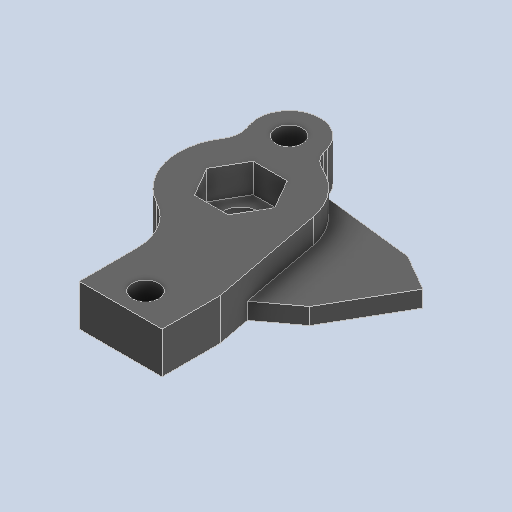
# Autodesk Inventor part: screw_lift_under
Saved by Autodesk Inventor 2024.1 (Build 281209000, 209)
## iProperties
Created: 2025-01-18
Part Number: screw_lift_under
Material: 一般
Document SubType Name: Modeling
Designer: hibik
Density: 1 g/cm^3
Appearance: 既定
Author: hibik
Autodesk Inventor part; units mm, degrees
ref_plane "YZ Plane" through (0, 0, 0) normal (1, 0, 0) x (0, 1, 0)
ref_plane "XZ Plane" through (0, 0, 0) normal (0, 1, 0) x (-1, 0, 0)
ref_plane "XY Plane" through (0, 0, 0) normal (0, 0, 1) x (1, 0, 0)
sketch "スケッチ1" plane through (0, 0, 0) normal (0, 1, 0) x (-1, 0, 0)
  line L0 (0, 0) -> (-19.1969, -33.25)
  line L1 (-19.1969, -33.25) -> (-10.9697, -38)
  line L2 (-10.9697, -38) -> (10.656, -38)
  line L3 (23.0438, 0) -> (-50.7627, 0) projected
  circle A0 centre (0, -50.5) radius 12.5
  line L4 (-19.1969, -33.25) -> (-30, -51.9615)
  line L5 (-30, -51.9615) -> (-40.219, -46.0616) construction
  line L6 (-30, -51.9615) -> (-24.5152, -61.4615)
  line L7 (-10.9697, -38) -> (-24.5152, -61.4615)
  line L8 (-24.5152, -61.4615) -> (-14.7652, -44.574)
  line L9 (-14.7652, -44.574) -> (-9.2226, -47.774)
  line L10 (-9.2226, -47.774) -> (-18.9726, -64.6615)
  line L11 (-18.9726, -64.6615) -> (-24.5152, -61.4615)
  line L12 (-10, -38) -> (-10, -31)
  line L13 (-10, -31) -> (0, -31)
  line L14 (0, -31) -> (0, -38)
  line L15 (2.0496, -46.95) -> (4.0992, -50.5)
  line L16 (4.0992, -50.5) -> (2.0496, -54.05)
  line L17 (2.0496, -54.05) -> (-2.0496, -54.05)
  line L18 (-2.0496, -54.05) -> (-4.0992, -50.5)
  line L19 (-4.0992, -50.5) -> (-2.0496, -46.95)
  line L20 (-2.0496, -46.95) -> (2.0496, -46.95)
  circle A1 centre (0, -50.5) radius 7.5
  arc A2 (0, -38) -> (3.5294, -43.8824) centre (6.6667, -38) ccw
  line L21 (-10, -38) -> (-7.3691, -51.8953)
  line L22 (-14.2226, -56.4343) -> (-18.5527, -53.9343)
  line L23 (-18.5527, -53.9343) -> (-13.5527, -45.274)
  line L24 (-13.5527, -45.274) -> (-9.2226, -47.774)
  line L25 (-9.2226, -47.774) -> (-14.2226, -56.4343)
  line L26 (-13.5527, -45.274) -> (-9.2294, -42.0698)
  line L27 (-14.2226, -56.4343) -> (-0.8456, -57.9522)
  dimension "d0" = 38
  dimension "d1" = 60
  dimension "d2" = 9.5
  dimension "d3" = 25
  dimension "d4" = 60
  dimension "d5" = 60
  dimension "d6" = 19.5
  dimension "d7" = 6.4
  dimension "d8" = 10
  dimension "d9" = 7
  dimension "d10" = 7.1
  dimension "d11" = 15
  dimension "d12" = 5
  dimension "d13" = 10
  constraints: 54 end point, 7 point on circle, 5 parallel, 5 perpendicular, 5 point on line, 5 tangent, 3 centre point, 3 horizontal, 2 coincident, 2 collinear, 2 vertical, 1 vertical alignment, 13 other
  measures "d0" distance from line of L0.start L2
  measures "d1" angle of L3 L0
  measures "d2" distance from line of L1.end L0
  measures "d3" diameter of A0
  measures "d4" distance from line of L0.start L5
  measures "d5" angle of L4 L6
  measures "d6" distance between parallel lines of L11 L9
  measures "d7" distance between parallel lines of L7 L10
  measures "d8" distance of L12.end L13.end
  measures "d9" distance between parallel lines of L2 L13
  measures "d10" distance between parallel lines of L20 L17
  measures "d11" diameter of A1
  measures "d12" distance between parallel lines of L25 L23
  measures "d13" distance between parallel lines of L9 L22
extrude "押し出し1" add sketch "スケッチ1" along normal blind 2 contours L12 L13 L14 L2 | L2 A0 L21 | A2 A1 L21 A0 | L21 A1 L27 A0 L10 L9 | A0 L9 L26 | L9 A0 L10 L22 L23 | A1 | L9 L10 A0 | L10 A0 L27
extrude "押し出し3" add sketch "スケッチ1" along normal blind 5 contours L12 L13 L14 L2 | L2 A0 L21 | A2 A1 L21 A0 | A1
sketch "スケッチ2" plane through (0, 0, 0) normal (0, -1, 0) x (1, 0, 0)
  line L0 (-2.0496, -46.95) -> (-4.0992, -50.5) projected
  line L1 (2.0496, -46.95) -> (-2.0496, -46.95) projected
  line L2 (4.0992, -50.5) -> (2.0496, -46.95) projected
  line L3 (2.0496, -54.05) -> (4.0992, -50.5) projected
  line L4 (-2.0496, -54.05) -> (2.0496, -54.05) projected
  line L5 (-4.0992, -50.5) -> (-2.0496, -54.05) projected
  circle A0 centre (0, -50.5) radius 3.55
  circle A1 centre (0, -50.5) radius 2.15
  point P0 (0, 0)
  dimension "d16" = 4.3
  constraints: 3 tangent, 2 centre point, 1 coincident
  measures "d16" diameter of A1
extrude "押し出し2" add sketch "スケッチ2" against normal blind 1.5
sketch "スケッチ3" plane through (0, 5, 0) normal (0, 1, 0) x (1, 0, 0)
  arc A0 (7.3691, 51.8953) -> (-3.5294, 43.8824) centre (0, 50.5) ccw projected
  circle A1 centre (0, 50.5) radius 12.5
  circle A2 centre (-2.5376, 58.874) radius 1.6
  circle A3 centre (-2.5376, 58.874) radius 3.75
  line L0 (-6.1264, 57.7864) -> (1.0513, 59.9615)
  line L1 (1.0513, 59.9615) -> (1.7052, 57.8036)
  line L2 (1.7052, 57.8036) -> (-5.4725, 55.6285)
  line L3 (-5.4725, 55.6285) -> (-6.1264, 57.7864)
  line L4 (0, 50.5) -> (-1.8837, 56.7161)
  circle A4 centre (5, 34) radius 1.6
  line L5 (10, 31) -> (10, 38) projected
  line L6 (10, 37) -> (0, 37)
  line L7 (0, 31) -> (10, 31) projected
  line L8 (0, 37) -> (10, 31) construction
  line L9 (10, 37) -> (0, 31) construction
  line L10 (0, 50.5) -> (5, 34)
  line L11 (10, 31) -> (10, 38) projected
  line L12 (0, 38) -> (0, 31) projected
  point P0 (0, 0)
  point P1 (1.7052, 57.8036)
  point P2 (-1.0063, 59.338)
  point P3 (-4.0688, 58.41)
  dimension "d21" = 25
  dimension "d22" = 3.2
  dimension "d23" = 7.5
  dimension "d24" = 3.2
  dimension "d33" = 1
  constraints: 18 end point, 4 midpoint, 3 centre point, 3 point on circle, 2 coincident, 2 parallel, 2 perpendicular, 2 point on line, 1 collinear, 1 horizontal, 1 vertical alignment, 2 other
  measures "d22" diameter of A2
  measures "d23" diameter of A3
  measures "d24" diameter of A4
  measures "d33" distance from line of L5.end L6
extrude "押し出し4" add sketch "スケッチ3" against normal up to surface (5 mm away) contours A0 A3 L1 | A3 L0 A2 | A0 A2 L0 A3 | A0 A3 L0 A2 | A3 A0 L3
extrude "押し出し5" cut sketch "スケッチ3" against normal through all contours A2 A0 | A0 A2 L0 | A4
fillet "フィレット1" radius 3 2 edges at (1.7052, 3.5, -57.8036) (-5.4725, 2.5, -55.6285)
sketch "スケッチ4" plane through (0, 0, 0) normal (0, -1, 0) x (1, 0, 0)
  circle A0 centre (-2.5376, -58.874) radius 1.6 projected
  line L0 (-5.8285, -58.874) -> (-4.183, -56.024)
  line L1 (-4.183, -56.024) -> (-0.8921, -56.024)
  line L2 (-0.8921, -56.024) -> (0.7533, -58.874)
  line L3 (0.7533, -58.874) -> (-0.8921, -61.724)
  line L4 (-0.8921, -61.724) -> (-4.183, -61.724)
  line L5 (-4.183, -61.724) -> (-5.8285, -58.874)
  point P0 (0, 0)
  point P1 (-3.1634, -57.3002)
  point P2 (-1.4067, -57.8669)
  dimension "d30" = 5.7
  constraints: 12 end point, 1 coincident, 1 horizontal, 14 other
  measures "d30" distance between parallel lines of L4 L1
extrude "押し出し6" cut sketch "スケッチ4" against normal blind 2
